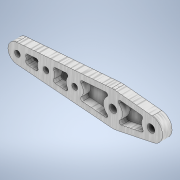
# Autodesk Inventor part: カウンター 取り付け根元
Saved by Autodesk Inventor 2020.2 (Build 242310000, 310)
## iProperties
Created: 2020-05-03
Part Number: カウンター 取り付け根元
Material: アルミニウム 7075
Document SubType Name: Modeling
Designer: mozar
Density: 2.81 g/cm^3
Appearance: サテン - ブラシ仕上げ 重厚
Mass: 11.2849 g
Surface Area: 38.3357 cm^2
Volume: 4.01597 cm^3
Author: mozar
Autodesk Inventor part; units mm, degrees
ref_plane "YZ Plane" through (0, 0, 0) normal (1, 0, 0) x (0, 1, 0)
ref_plane "XZ Plane" through (0, 0, 0) normal (0, 1, 0) x (-1, 0, 0)
ref_plane "XY Plane" through (0, 0, 0) normal (0, 0, 1) x (1, 0, 0)
sketch "スケッチ1" plane through (0, 0, 0) normal (0, 0, 1) x (1, 0, 0)
  circle A0 centre (-137.4781, 108.715) radius 1.5
  circle A1 centre (-137.4781, 108.715) radius 4
  circle A2 centre (-84.8339, 108.085) radius 1.5
  circle A3 centre (-84.8339, 108.085) radius 4
  arc A4 (-118.9473, 71.1234) -> (-117.731, 71.3822) centre (-118.5021, 72.0189) ccw
  arc A5 (-114.6003, 73.9072) -> (-117.731, 71.3822) centre (-110, 65) ccw
  arc A6 (-114.6003, 73.9072) -> (-114.0897, 75.0411) centre (-115.0592, 74.7957) ccw
  line L0 (-114.0897, 75.0411) -> (-119.3334, 95.7508)
  arc A7 (-119.3334, 95.7508) -> (-120.0808, 96.4804) centre (-120.3028, 95.5054) ccw
  arc A8 (-121.7309, 97.2305) -> (-120.0808, 96.4804) centre (-119.0818, 100.8681) ccw
  arc A9 (-121.7309, 97.2305) -> (-122.772, 97.314) centre (-122.3196, 96.4222) ccw
  line L1 (-122.772, 97.314) -> (-145.177, 85.9475)
  arc A10 (-145.177, 85.9475) -> (-145.1697, 84.1603) centre (-144.7246, 85.0557) ccw
  line L2 (-145.1697, 84.1603) -> (-118.9473, 71.1234)
  arc A11 (-111.1815, 75.7775) -> (-110.1929, 75.0231) centre (-110.2121, 76.023) ccw
  arc A12 (-100.6814, 68.6965) -> (-110.1929, 75.0231) centre (-110, 65) ccw
  arc A13 (-100.6814, 68.6965) -> (-99.6035, 68.0763) centre (-99.7518, 69.0652) ccw
  line L3 (-99.6035, 68.0763) -> (-77.0424, 71.4604)
  arc A14 (-77.0424, 71.4604) -> (-76.6709, 73.3036) centre (-77.1908, 72.4494) ccw
  line L4 (-76.6709, 73.3036) -> (-114.6373, 96.4076)
  arc A15 (-114.6373, 96.4076) -> (-116.1266, 95.3079) centre (-115.1572, 95.5533) ccw
  line L5 (-116.1266, 95.3079) -> (-111.1815, 75.7775)
  circle A16 centre (-150.2948, 85.0332) radius 1.5
  arc A17 (-124.1293, 99.9894) -> (-123.5818, 100.8788) centre (-124.5818, 100.8812) ccw
  arc A18 (-114.5944, 100.5318) -> (-123.5818, 100.8788) centre (-119.0818, 100.8681) ccw
  arc A19 (-114.5944, 100.5318) -> (-114.117, 99.6028) centre (-113.5972, 100.457) ccw
  line L6 (-114.117, 99.6028) -> (-73.4052, 74.8281)
  arc A20 (-73.4052, 74.8281) -> (-72.3608, 74.831) centre (-72.8854, 75.6824) ccw
  arc A21 (-73.6605, 68.3826) -> (-72.3608, 74.831) centre (-70, 71) ccw
  arc A22 (-73.6605, 68.3826) -> (-74.6223, 68.7899) centre (-74.4739, 67.8009) ccw
  line L7 (-74.6223, 68.7899) -> (-99.1585, 65.1094)
  arc A23 (-99.1585, 65.1094) -> (-100.0069, 64.2003) centre (-99.0101, 64.1205) ccw
  arc A24 (-119.755, 67.3111) -> (-100.0069, 64.2003) centre (-110, 65) ccw
  arc A25 (-119.755, 67.3111) -> (-120.2828, 68.4371) centre (-120.728, 67.5417) ccw
  line L8 (-120.2828, 68.4371) -> (-147.0852, 81.7623)
  arc A26 (-147.0852, 81.7623) -> (-148.0833, 81.7001) centre (-147.5304, 80.8669) ccw
  arc A27 (-148.1104, 88.384) -> (-148.0833, 81.7001) centre (-150.2948, 85.0332) ccw
  arc A28 (-148.1104, 88.384) -> (-147.1118, 88.3299) centre (-147.5643, 89.2217) ccw
  line L9 (-147.1118, 88.3299) -> (-124.1293, 99.9894)
  circle A29 centre (-110, 65) radius 7.025
  circle A30 centre (-119.0818, 100.8681) radius 1.5
  circle A31 centre (-70, 71) radius 1.5
  line L10 (-330.4, 95) -> (-110, 65)
  circle A32 centre (-156.4432, 91.1623) radius 4
  circle A33 centre (-136.4706, 92.2091) radius 4
  line L11 (0, 0) -> (-155.7948, 0)
  line L12 (-329.0512, 104.9086) -> (-108.6513, 74.9086)
  circle A34 centre (-156.4432, 91.1623) radius 9
  circle A35 centre (-136.4706, 92.2091) radius 6
  line L13 (-156.4432, 91.1623) -> (-136.4706, 92.2091)
  circle A36 centre (-110, 65) radius 65
  circle A37 centre (-191.4432, 91.1623) radius 5
  line L14 (-191.4432, 91.1623) -> (-156.4432, 91.1623)
  line L15 (-191.4432, 91.1623) -> (-206.4432, 91.1623)
  circle A38 centre (-206.4432, 91.1623) radius 5
  line L16 (-206.4432, 91.1623) -> (-221.4432, 91.1623)
  circle A39 centre (-221.4432, 91.1623) radius 5
  line L17 (-221.4432, 91.1623) -> (-236.4432, 91.1623)
  circle A40 centre (-236.4432, 91.1623) radius 5
  line L18 (-206.8432, 96.1463) -> (-157.1632, 100.1335)
  line L19 (-206.8432, 86.1784) -> (-157.1632, 82.1912)
  line L20 (-135.8823, 98.1801) -> (-155.5608, 100.119)
  line L21 (-154.6294, 82.347) -> (-135.2614, 86.3322)
  circle A41 centre (-206.4432, 91.1623) radius 1.5
  circle A42 centre (-191.4432, 91.1623) radius 1.5
  point P0 (-202.8118, 87.7254)
  point P1 (-169.3241, 83.1672)
  point P2 (-153.5101, 82.6537)
  point P3 (-153.4601, 82.5876)
  point P4 (-191.3368, 86.1635)
  point P5 (-192.8818, 86.3738)
  dimension "d0" = 8
  dimension "d1" = 8
  dimension "d2" = 95
  dimension "d3" = 7.751
  dimension "d4" = 10
  dimension "d5" = 18
  dimension "d6" = 12
  dimension "d7" = 20
  dimension "d8" = 3
  dimension "d9" = 130
  dimension "d10" = 10
  dimension "d11" = 35
  dimension "d12" = 15
  dimension "d13" = 10
  dimension "d14" = 15
  dimension "d15" = 10
  dimension "d16" = 15
  dimension "d17" = 10
  dimension "d18" = 3
  dimension "d19" = 3
  constraints: 56 point on circle, 44 end point, 43 centre point, 9 tangent, 8 coincident, 6 horizontal, 1 parallel, 11 other
  measures "d0" diameter of A32
  measures "d1" diameter of A33
  measures "d2" distance from line of L11 L10.start
  measures "d3" angle of L11 L10
  measures "d4" distance between parallel lines of L10 L12
  measures "d5" diameter of A34
  measures "d6" diameter of A35
  measures "d7" distance of A32.centre A33.centre
  measures "d8" angle of L11 L13
  measures "d9" diameter of A36
  measures "d10" diameter of A37
  measures "d11" distance of L14.start L13.start
  measures "d12" distance of L14.start L15.end
  measures "d13" diameter of A38
  measures "d14" distance of L16.start L16.end
  measures "d15" diameter of A39
  measures "d16" distance of L17.start L17.end
  measures "d17" diameter of A40
  measures "d18" diameter of A41
  measures "d19" diameter of A42
extrude "押し出し1" add sketch "スケッチ1" against normal blind 5 contours L21 A27 A34 A16 A28 L9 A35 L1 A10 | A10 L1 A35 L21 | L19 A36 L12 | L12 A36 L14 A34 L19 | A35 L1 A33 | A36 L19 A38 L12 A37 | L12 A37 L14 A36 | A34 L14 A32 L13 A28 A27 | A35 L9 A33 L1 | A27 A28 A34 A16 | A37 L12 | L12 A37 L15 A42 L14 | L14 A37 L15 A38 L18 A36 | A36 L18 A34 L14 | A38 L12 | A34 L13 A32 L14 | A33 L9 L1 | L1 A33 | A35 L13 A33 L9 | L9 A28 A34 L13 A35 | A34 A16 | A16 A34 | L1 A33 L9 A35 | L12 A38 L15 A37 | L14 A42 L15 A37 | A38 L16 A41 L15 L12 | L14 L13 A32 | A32 L13 L14 | A33 L13 L9 | L13 A34 L20 A35 | A35 L9 A33 L13 | A38 L15 A41 L16 | L9 L13 A33
hole "穴1" at (-156.4432, 91.1623, 0) at (-136.4706, 92.2091, 0) direction (0, 0, -1) diameter 4 depth 12 tip angle 118
sketch "スケッチ2" plane through (0, 0, 0) normal (0, 0, 1) x (1, 0, 0)
  circle A0 centre (-156.4432, 91.1623) radius 2 projected
  circle A1 centre (-136.4706, 92.2091) radius 2 projected
  circle A2 centre (-191.4432, 91.1623) radius 1.5 projected
  circle A3 centre (-206.4432, 91.1623) radius 1.5 projected
  arc A4 (-157.1632, 82.1912) -> (-153.5101, 82.6537) centre (-156.4432, 91.1623) ccw projected
  line L0 (-157.1632, 82.1912) -> (-206.8432, 86.1784) projected
  arc A5 (-206.8432, 96.1463) -> (-206.8432, 86.1784) centre (-206.4432, 91.1623) ccw projected
  line L1 (-206.8432, 96.1463) -> (-157.1632, 100.1335) projected
  arc A6 (-155.5608, 100.119) -> (-157.1632, 100.1335) centre (-156.4432, 91.1623) ccw projected
  line L2 (-155.5608, 100.119) -> (-135.8823, 98.1801) projected
  arc A7 (-135.2614, 86.3322) -> (-135.8823, 98.1801) centre (-136.4706, 92.2091) ccw projected
  line L3 (-135.2614, 86.3322) -> (-153.4601, 82.5876) projected
  arc A8 (-153.5101, 82.6537) -> (-153.4601, 82.5876) centre (-150.2948, 85.0332) ccw projected
  line L4 (-156.9232, 97.1431) -> (-206.6032, 93.1559)
  arc A9 (-206.6032, 93.1559) -> (-206.6032, 89.1687) centre (-206.4432, 91.1623) ccw
  line L5 (-206.6032, 89.1687) -> (-156.9232, 85.1816)
  arc A10 (-156.9232, 85.1816) -> (-155.234, 85.2855) centre (-156.4432, 91.1623) ccw
  line L6 (-155.234, 85.2855) -> (-135.866, 89.2706)
  arc A11 (-135.866, 89.2706) -> (-136.1765, 95.1946) centre (-136.4706, 92.2091) ccw
  line L7 (-136.1765, 95.1946) -> (-155.8549, 97.1334)
  arc A12 (-155.8549, 97.1334) -> (-156.9232, 97.1431) centre (-156.4432, 91.1623) ccw
  circle A13 centre (-206.4432, 91.1623) radius 4.5
  circle A14 centre (-191.4432, 91.1623) radius 4.5
  circle A15 centre (-156.4432, 91.1623) radius 5
  circle A16 centre (-136.4706, 92.2091) radius 5
  circle A17 centre (-160.1492, 95.881) radius 1
  circle A18 centre (-152.6523, 95.813) radius 1
  circle A19 centre (-152.187, 86.9334) radius 1
  circle A20 centre (-160.1492, 86.4437) radius 1
  point P0 (0, 0)
  point P1 (-151.9854, 85.9539)
  point P2 (-139.7839, 88.4645)
  point P3 (-140.1572, 95.5868)
  point P4 (-152.5543, 96.8082)
  point P5 (-153.2841, 95.0379)
  point P6 (-152.8963, 87.6382)
  point P7 (-159.5315, 87.2301)
  point P8 (-159.5315, 95.0945)
  point P9 (-160.2292, 96.8778)
  point P10 (-188.5455, 94.6052)
  point P11 (-188.5455, 87.7195)
  point P12 (-160.2292, 85.4469)
  point P13 (-194.8529, 88.2257)
  point P14 (-194.8529, 94.099)
  point P15 (-202.585, 93.4784)
  point P16 (-202.585, 88.8463)
  dimension "d29" = 3
  dimension "d30" = 3
  dimension "d31" = 3
  dimension "d32" = 3
  dimension "d33" = 3
  dimension "d34" = 2
  dimension "d35" = 2
  dimension "d36" = 2
  dimension "d37" = 2
  constraints: 12 centre point, 8 end point, 8 point on circle, 8 tangent, 7 other
  measures "d29" distance between parallel lines of L4 L1
  measures "d30" radial gap between concentric circles of A3 A13
  measures "d31" radial gap between concentric circles of A2 A14
  measures "d32" radial gap between concentric circles of A0 A15
  measures "d33" radial gap between concentric circles of A1 A16
  measures "d34" diameter of A17
  measures "d35" diameter of A18
  measures "d36" diameter of A19
  measures "d37" diameter of A20
extrude "押し出し2" cut sketch "スケッチ2" against normal blind 4 contours A17 A15 A20 L5 A14 L4 | A17 | L7 A16 L6 A19 A15 A18 | A18 | A14 L5 A13 L4 | A20 | A19
fillet "フィレット1" radius 1 8 edges at (-202.585, 93.4784, -2) (-202.585, 88.8463, -2) (-194.8529, 94.099, -2) (-194.8529, 88.2257, -2) (-188.5455, 94.6052, -2) (-188.5455, 87.7195, -2) (-140.1572, 95.5868, -2) (-139.7839, 88.4645, -2)
sketch "スケッチ3" plane through (0, 0, 0) normal (0, 0, 1) x (1, 0, 0)
  arc A0 (-202.0979, 89.9928) -> (-201.2122, 88.7361) centre (-201.1322, 89.7329) ccw projected
  line L0 (-201.2122, 88.7361) -> (-196.7239, 88.3759) projected
  arc A1 (-196.7239, 88.3759) -> (-195.6983, 89.6981) centre (-196.6439, 89.3727) ccw projected
  arc A2 (-195.6983, 92.6266) -> (-195.6983, 89.6981) centre (-191.4432, 91.1623) ccw projected
  arc A3 (-195.6983, 92.6266) -> (-196.7239, 93.9488) centre (-196.6439, 92.952) ccw projected
  line L1 (-196.7239, 93.9488) -> (-201.2122, 93.5886) projected
  arc A4 (-201.2122, 93.5886) -> (-202.0979, 92.3319) centre (-201.1322, 92.5918) ccw projected
  arc A5 (-202.0979, 89.9928) -> (-202.0979, 92.3319) centre (-206.4432, 91.1623) ccw projected
  arc A6 (-152.8963, 87.6382) -> (-153.2841, 95.0379) centre (-156.4432, 91.1623) ccw projected
  arc A7 (-152.8963, 87.6382) -> (-151.9854, 85.9539) centre (-152.187, 86.9334) ccw projected
  line L2 (-151.9854, 85.9539) -> (-141.4068, 88.1305) projected
  arc A8 (-141.4068, 88.1305) -> (-140.752, 89.6265) centre (-141.6083, 89.11) ccw projected
  arc A9 (-140.9985, 94.3299) -> (-140.752, 89.6265) centre (-136.4706, 92.2091) ccw projected
  arc A10 (-140.9985, 94.3299) -> (-141.8061, 95.7493) centre (-141.9041, 94.7541) ccw projected
  line L3 (-141.8061, 95.7493) -> (-152.5543, 96.8082) projected
  arc A11 (-152.5543, 96.8082) -> (-153.2841, 95.0379) centre (-152.6523, 95.813) ccw projected
  arc A12 (-159.5315, 95.0945) -> (-159.5315, 87.2301) centre (-156.4432, 91.1623) ccw projected
  arc A13 (-159.5315, 95.0945) -> (-160.2292, 96.8778) centre (-160.1492, 95.881) ccw projected
  line L4 (-160.2292, 96.8778) -> (-186.6745, 94.7553) projected
  arc A14 (-186.6745, 94.7553) -> (-187.4761, 93.2865) centre (-186.5945, 93.7586) ccw projected
  arc A15 (-187.4761, 89.0382) -> (-187.4761, 93.2865) centre (-191.4432, 91.1623) ccw projected
  arc A16 (-187.4761, 89.0382) -> (-186.6745, 87.5693) centre (-186.5945, 88.5661) ccw projected
  line L5 (-186.6745, 87.5693) -> (-160.2292, 85.4469) projected
  arc A17 (-160.2292, 85.4469) -> (-159.5315, 87.2301) centre (-160.1492, 86.4437) ccw projected
  circle A18 centre (-156.4432, 91.1623) radius 2 projected
  circle A19 centre (-136.4706, 92.2091) radius 2 projected
  circle A20 centre (-191.4432, 91.1623) radius 1.5 projected
  circle A21 centre (-206.4432, 91.1623) radius 1.5 projected
  arc A22 (-157.1632, 82.1912) -> (-153.5101, 82.6537) centre (-156.4432, 91.1623) ccw projected
  line L6 (-157.1632, 82.1912) -> (-206.8432, 86.1784) projected
  arc A23 (-206.8432, 96.1463) -> (-206.8432, 86.1784) centre (-206.4432, 91.1623) ccw projected
  line L7 (-206.8432, 96.1463) -> (-157.1632, 100.1335) projected
  arc A24 (-155.5608, 100.119) -> (-157.1632, 100.1335) centre (-156.4432, 91.1623) ccw projected
  line L8 (-155.5608, 100.119) -> (-135.8823, 98.1801) projected
  arc A25 (-135.2614, 86.3322) -> (-135.8823, 98.1801) centre (-136.4706, 92.2091) ccw projected
  line L9 (-135.2614, 86.3322) -> (-153.4601, 82.5876) projected
  arc A26 (-153.5101, 82.6537) -> (-153.4601, 82.5876) centre (-150.2948, 85.0332) ccw projected
  circle A27 centre (-206.4432, 91.1623) radius 1.5 projected
  circle A28 centre (-156.4432, 91.1623) radius 2 projected
  line L10 (-206.4432, 91.1623) -> (-156.4432, 91.1623)
  circle A29 centre (-176.4432, 91.1623) radius 1.5
  circle A30 centre (-176.4432, 91.1623) radius 4.5
  circle A31 centre (-161.4432, 91.1623) radius 4.5
  circle A32 centre (-161.4432, 91.1623) radius 1.5
  point P0 (0, 0)
  dimension "d41" = 3
  dimension "d42" = 3
  dimension "d43" = 15
  dimension "d44" = 9
  dimension "d45" = 3
  dimension "d46" = 15
  constraints: 4 centre point, 2 end point, 2 point on line, 1 coincident, 1 horizontal
  measures "d41" diameter of A29
  measures "d42" radial gap between concentric circles of A29 A30
  measures "d43" distance of A29.centre A2.centre
  measures "d44" diameter of A31
  measures "d45" diameter of A32
  measures "d46" distance of A29.centre A31.centre
extrude "押し出し3" add sketch "スケッチ3" against normal blind 5 contours A30 L10 A29 L4 | L4 A30 | A30 L5 L10 A29 | A30 L5
fillet "フィレット2" radius 1 4 edges at (-175.8548, 95.6237, -2) (-177.7356, 95.4728, -2) (-175.8548, 86.701, -2) (-177.7356, 86.8519, -2)
sketch "スケッチ4" plane through (0, 0, 0) normal (0, 0, 1) x (1, 0, 0)
  arc A0 (-181.1046, 87.1223) -> (-180.1916, 88.6724) centre (-181.0246, 88.1191) ccw projected
  arc A1 (-180.1916, 93.6523) -> (-180.1916, 88.6724) centre (-176.4432, 91.1623) ccw projected
  arc A2 (-180.1916, 93.6523) -> (-181.1046, 95.2024) centre (-181.0246, 94.2056) ccw projected
  line L0 (-181.1046, 95.2024) -> (-186.6745, 94.7553) projected
  arc A3 (-186.6745, 94.7553) -> (-187.4761, 93.2865) centre (-186.5945, 93.7586) ccw projected
  arc A4 (-187.4761, 89.0382) -> (-187.4761, 93.2865) centre (-191.4432, 91.1623) ccw projected
  arc A5 (-187.4761, 89.0382) -> (-186.6745, 87.5693) centre (-186.5945, 88.5661) ccw projected
  line L1 (-186.6745, 87.5693) -> (-181.1046, 87.1223) projected
  circle A6 centre (-176.4432, 91.1623) radius 1.5 projected
  arc A7 (-202.0979, 89.9928) -> (-201.2122, 88.7361) centre (-201.1322, 89.7329) ccw projected
  line L2 (-201.2122, 88.7361) -> (-196.7239, 88.3759) projected
  arc A8 (-196.7239, 88.3759) -> (-195.6983, 89.6981) centre (-196.6439, 89.3727) ccw projected
  arc A9 (-195.6983, 92.6266) -> (-195.6983, 89.6981) centre (-191.4432, 91.1623) ccw projected
  arc A10 (-195.6983, 92.6266) -> (-196.7239, 93.9488) centre (-196.6439, 92.952) ccw projected
  line L3 (-196.7239, 93.9488) -> (-201.2122, 93.5886) projected
  arc A11 (-201.2122, 93.5886) -> (-202.0979, 92.3319) centre (-201.1322, 92.5918) ccw projected
  arc A12 (-202.0979, 89.9928) -> (-202.0979, 92.3319) centre (-206.4432, 91.1623) ccw projected
  arc A13 (-152.8963, 87.6382) -> (-153.2841, 95.0379) centre (-156.4432, 91.1623) ccw projected
  arc A14 (-152.8963, 87.6382) -> (-151.9854, 85.9539) centre (-152.187, 86.9334) ccw projected
  line L4 (-151.9854, 85.9539) -> (-141.4068, 88.1305) projected
  arc A15 (-141.4068, 88.1305) -> (-140.752, 89.6265) centre (-141.6083, 89.11) ccw projected
  arc A16 (-140.9985, 94.3299) -> (-140.752, 89.6265) centre (-136.4706, 92.2091) ccw projected
  arc A17 (-140.9985, 94.3299) -> (-141.8061, 95.7493) centre (-141.9041, 94.7541) ccw projected
  line L5 (-141.8061, 95.7493) -> (-152.5543, 96.8082) projected
  arc A18 (-152.5543, 96.8082) -> (-153.2841, 95.0379) centre (-152.6523, 95.813) ccw projected
  arc A19 (-159.5315, 95.0945) -> (-159.5315, 87.2301) centre (-156.4432, 91.1623) ccw projected
  arc A20 (-159.5315, 95.0945) -> (-160.2292, 96.8778) centre (-160.1492, 95.881) ccw projected
  line L6 (-160.2292, 96.8778) -> (-172.4859, 95.8941) projected
  arc A21 (-172.4859, 95.8941) -> (-173.1399, 94.2182) centre (-172.4059, 94.8973) ccw projected
  arc A22 (-173.1399, 88.1065) -> (-173.1399, 94.2182) centre (-176.4432, 91.1623) ccw projected
  arc A23 (-173.1399, 88.1065) -> (-172.4859, 86.4306) centre (-172.4059, 87.4274) ccw projected
  line L7 (-172.4859, 86.4306) -> (-160.2292, 85.4469) projected
  arc A24 (-160.2292, 85.4469) -> (-159.5315, 87.2301) centre (-160.1492, 86.4437) ccw projected
  circle A25 centre (-156.4432, 91.1623) radius 2 projected
  circle A26 centre (-136.4706, 92.2091) radius 2 projected
  circle A27 centre (-191.4432, 91.1623) radius 1.5 projected
  circle A28 centre (-206.4432, 91.1623) radius 1.5 projected
  arc A29 (-157.1632, 82.1912) -> (-153.5101, 82.6537) centre (-156.4432, 91.1623) ccw projected
  line L8 (-157.1632, 82.1912) -> (-206.8432, 86.1784) projected
  arc A30 (-206.8432, 96.1463) -> (-206.8432, 86.1784) centre (-206.4432, 91.1623) ccw projected
  line L9 (-206.8432, 96.1463) -> (-157.1632, 100.1335) projected
  arc A31 (-155.5608, 100.119) -> (-157.1632, 100.1335) centre (-156.4432, 91.1623) ccw projected
  line L10 (-155.5608, 100.119) -> (-135.8823, 98.1801) projected
  arc A32 (-135.2614, 86.3322) -> (-135.8823, 98.1801) centre (-136.4706, 92.2091) ccw projected
  line L11 (-135.2614, 86.3322) -> (-153.4601, 82.5876) projected
  arc A33 (-153.5101, 82.6537) -> (-153.4601, 82.5876) centre (-150.2948, 85.0332) ccw projected
  point P0 (0, 0)
hole "穴2" at (-176.4432, 91.1623, 0) direction (0, 0, -1) diameter 3 depth 12 tip angle 118
